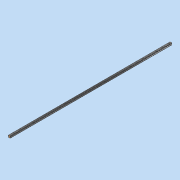
# Autodesk Inventor part: HGR20 THANH TRUOT
Saved by Autodesk Inventor 2021 (Build 250183000, 183)
## iProperties
Created: 2021-09-26
Part Number: HGR20 THANH TRUOT
Material: Generic
Document SubType Name: Modeling
Designer: 41601100
Density: 1 g/cm^3
Appearance: Default
Author: 41601100
Autodesk Inventor part; units mm, degrees
ref_plane "YZ Plane" through (0, 0, 0) normal (1, 0, 0) x (0, 1, 0)
ref_plane "XZ Plane" through (0, 0, 0) normal (0, 1, 0) x (-1, 0, 0)
ref_plane "XY Plane" through (0, 0, 0) normal (0, 0, 1) x (1, 0, 0)
sketch "Sketch1" plane through (0, 0, 0) normal (0, 0, 1) x (1, 0, 0)
  arc A0 (-9.7071, -9.6314) -> (-10, -10.3385) centre (-9, -10.3385) ccw
  line L0 (-10, -10.3385) -> (-10, -13)
  line L1 (-10, -13) -> (-9, -14)
  line L2 (-9, -14) -> (9, -14)
  line L3 (9, -14) -> (10, -13)
  line L4 (10, -13) -> (10, -10.3385)
  arc A1 (10, -10.3385) -> (9.7071, -9.6314) centre (9, -10.3385) ccw
  line L5 (9.7071, -9.6314) -> (6.8929, -6.8172)
  arc A2 (6.6, -6.1101) -> (6.8929, -6.8172) centre (7.6, -6.1101) ccw
  line L6 (6.6, -6.1101) -> (6.6, -4.5499)
  arc A3 (6.8929, -3.8428) -> (6.6, -4.5499) centre (7.6, -4.5499) ccw
  line L7 (6.8929, -3.8428) -> (7.6302, -3.1056)
  arc A4 (7.6302, -3.1056) -> (7.8468, -2.7675) centre (7.3529, -2.6895) ccw
  arc A5 (9.4318, -1.1825) -> (7.8468, -2.7675) centre (9.8106, -3.1463) ccw
  arc A6 (9.4318, -1.1825) -> (9.6906, -1.0451) centre (9.3371, -0.6915) ccw
  line L8 (9.6906, -1.0451) -> (9.8536, -0.8822)
  arc A7 (9.8536, -0.8822) -> (10, -0.5286) centre (9.5, -0.5286) ccw
  line L9 (10, -0.5286) -> (10, 0.5286)
  arc A8 (10, 0.5286) -> (9.8536, 0.8822) centre (9.5, 0.5286) ccw
  line L10 (9.8536, 0.8822) -> (9.6906, 1.0451)
  arc A9 (9.6906, 1.0451) -> (9.4224, 1.1941) centre (9.3254, 0.7036) ccw
  arc A10 (7.8482, 2.768) -> (9.4224, 1.1941) centre (9.8101, 3.1561) ccw
  arc A11 (7.8482, 2.768) -> (7.6325, 3.1032) centre (7.3547, 2.6875) ccw
  line L11 (7.6325, 3.1032) -> (7.2357, 3.5)
  line L12 (7.2357, 3.5) -> (-7.2357, 3.5)
  line L13 (-7.2357, 3.5) -> (-7.6325, 3.1032)
  arc A12 (-7.6325, 3.1032) -> (-7.8482, 2.768) centre (-7.3547, 2.6875) ccw
  arc A13 (-9.4224, 1.1941) -> (-7.8482, 2.768) centre (-9.8101, 3.1561) ccw
  arc A14 (-9.4224, 1.1941) -> (-9.6906, 1.0451) centre (-9.3254, 0.7036) ccw
  line L14 (-9.6906, 1.0451) -> (-9.8536, 0.8822)
  arc A15 (-9.8536, 0.8822) -> (-10, 0.5286) centre (-9.5, 0.5286) ccw
  line L15 (-10, 0.5286) -> (-10, -0.5286)
  arc A16 (-10, -0.5286) -> (-9.8536, -0.8822) centre (-9.5, -0.5286) ccw
  line L16 (-9.8536, -0.8822) -> (-9.6906, -1.0451)
  arc A17 (-9.6906, -1.0451) -> (-9.4318, -1.1825) centre (-9.3371, -0.6915) ccw
  arc A18 (-7.8468, -2.7675) -> (-9.4318, -1.1825) centre (-9.8106, -3.1463) ccw
  arc A19 (-7.8468, -2.7675) -> (-7.6302, -3.1056) centre (-7.3529, -2.6895) ccw
  line L17 (-7.6302, -3.1056) -> (-6.8929, -3.8428)
  arc A20 (-6.6, -4.5499) -> (-6.8929, -3.8428) centre (-7.6, -4.5499) ccw
  line L18 (-6.6, -4.5499) -> (-6.6, -6.1101)
  arc A21 (-6.8929, -6.8172) -> (-6.6, -6.1101) centre (-7.6, -6.1101) ccw
  line L19 (-6.8929, -6.8172) -> (-9.7071, -9.6314)
  point P0 (0, 0)
  point P1 (0, 0)
  constraints: 44 point on circle, 40 end point, 22 centre point
extrude "Extrusion1" add sketch "Sketch1" along normal blind 1500
sketch "Sketch2" plane through (-7.2357, 3.5, 1500) normal (0, 1, 0) x (1, 0, 0)
  line L0 (14.4714, 1500) -> (0, 1500) projected
  line L1 (0, 1500) -> (0, 0) projected
  line L2 (14.4714, 0) -> (0, 0) projected
  line L3 (14.4714, 1500) -> (14.4714, 0) projected
  circle A0 centre (7.2357, 1480) radius 4.75
  circle A1 centre (7.2357, 1480) radius 3
  circle A2 centre (7.2357, 1420) radius 4.75
  circle A3 centre (7.2357, 1420) radius 3
  circle A4 centre (7.2357, 1360) radius 4.75
  circle A5 centre (7.2357, 1360) radius 3
  circle A6 centre (7.2357, 1300) radius 4.75
  circle A7 centre (7.2357, 1300) radius 3
  circle A8 centre (7.2357, 1240) radius 4.75
  circle A9 centre (7.2357, 1240) radius 3
  circle A10 centre (7.2357, 1180) radius 4.75
  circle A11 centre (7.2357, 1180) radius 3
  circle A12 centre (7.2357, 1120) radius 4.75
  circle A13 centre (7.2357, 1120) radius 3
  circle A14 centre (7.2357, 1060) radius 4.75
  circle A15 centre (7.2357, 1060) radius 3
  circle A16 centre (7.2357, 1000) radius 4.75
  circle A17 centre (7.2357, 1000) radius 3
  circle A18 centre (7.2357, 940) radius 4.75
  circle A19 centre (7.2357, 940) radius 3
  circle A20 centre (7.2357, 880) radius 4.75
  circle A21 centre (7.2357, 880) radius 3
  circle A22 centre (7.2357, 820) radius 4.75
  circle A23 centre (7.2357, 820) radius 3
  circle A24 centre (7.2357, 760) radius 4.75
  circle A25 centre (7.2357, 760) radius 3
  circle A26 centre (7.2357, 700) radius 4.75
  circle A27 centre (7.2357, 700) radius 3
  circle A28 centre (7.2357, 640) radius 4.75
  circle A29 centre (7.2357, 640) radius 3
  circle A30 centre (7.2357, 580) radius 4.75
  circle A31 centre (7.2357, 580) radius 3
  circle A32 centre (7.2357, 520) radius 4.75
  circle A33 centre (7.2357, 520) radius 3
  circle A34 centre (7.2357, 460) radius 4.75
  circle A35 centre (7.2357, 460) radius 3
  circle A36 centre (7.2357, 400) radius 4.75
  circle A37 centre (7.2357, 400) radius 3
  circle A38 centre (7.2357, 340) radius 4.75
  circle A39 centre (7.2357, 340) radius 3
  circle A40 centre (7.2357, 280) radius 4.75
  circle A41 centre (7.2357, 280) radius 3
  circle A42 centre (7.2357, 220) radius 4.75
  circle A43 centre (7.2357, 220) radius 3
  circle A44 centre (7.2357, 160) radius 4.75
  circle A45 centre (7.2357, 160) radius 3
  circle A46 centre (7.2357, 100) radius 4.75
  circle A47 centre (7.2357, 100) radius 3
  circle A48 centre (7.2357, 40) radius 4.75
  circle A49 centre (7.2357, 40) radius 3
  point P0 (7.2357, 1500)
  dimension "d3" = 9.5
  dimension "d4" = 6
  dimension "d6" = 9.5
  dimension "d7" = 6
  dimension "d9" = 9.5
  dimension "d10" = 6
  dimension "d12" = 9.5
  dimension "d13" = 6
  dimension "d15" = 9.5
  dimension "d16" = 6
  dimension "d18" = 9.5
  dimension "d19" = 6
  dimension "d21" = 9.5
  dimension "d22" = 6
  dimension "d24" = 9.5
  dimension "d25" = 6
  dimension "d27" = 9.5
  dimension "d28" = 6
  dimension "d30" = 9.5
  dimension "d31" = 6
  dimension "d33" = 9.5
  dimension "d34" = 6
  dimension "d36" = 9.5
  dimension "d37" = 6
  dimension "d39" = 9.5
  dimension "d40" = 6
  dimension "d42" = 9.5
  dimension "d43" = 6
  dimension "d45" = 9.5
  dimension "d46" = 6
  dimension "d48" = 9.5
  dimension "d49" = 6
  dimension "d51" = 9.5
  dimension "d52" = 6
  dimension "d54" = 9.5
  dimension "d55" = 6
  dimension "d57" = 9.5
  dimension "d58" = 6
  dimension "d60" = 9.5
  dimension "d61" = 6
  dimension "d63" = 9.5
  dimension "d64" = 6
  dimension "d66" = 9.5
  dimension "d67" = 6
  dimension "d69" = 9.5
  dimension "d70" = 6
  dimension "d72" = 9.5
  dimension "d73" = 6
  dimension "d75" = 9.5
  dimension "d76" = 6
  constraints: 50 centre point, 25 coincident
  measures "d3" diameter of A0
  measures "d4" diameter of A1
  measures "d6" diameter of A2
  measures "d7" diameter of A3
  measures "d9" diameter of A4
  measures "d10" diameter of A5
  measures "d12" diameter of A6
  measures "d13" diameter of A7
  measures "d15" diameter of A8
  measures "d16" diameter of A9
  measures "d18" diameter of A10
  measures "d19" diameter of A11
  measures "d21" diameter of A12
  measures "d22" diameter of A13
  measures "d24" diameter of A14
  measures "d25" diameter of A15
  measures "d27" diameter of A16
  measures "d28" diameter of A17
  measures "d30" diameter of A18
  measures "d31" diameter of A19
  measures "d33" diameter of A20
  measures "d34" diameter of A21
  measures "d36" diameter of A22
  measures "d37" diameter of A23
  measures "d39" diameter of A24
  measures "d40" diameter of A25
  measures "d42" diameter of A26
  measures "d43" diameter of A27
  measures "d45" diameter of A28
  measures "d46" diameter of A29
  measures "d48" diameter of A30
  measures "d49" diameter of A31
  measures "d51" diameter of A32
  measures "d52" diameter of A33
  measures "d54" diameter of A34
  measures "d55" diameter of A35
  measures "d57" diameter of A36
  measures "d58" diameter of A37
  measures "d60" diameter of A38
  measures "d61" diameter of A39
  measures "d63" diameter of A40
  measures "d64" diameter of A41
  measures "d66" diameter of A42
  measures "d67" diameter of A43
  measures "d69" diameter of A44
  measures "d70" diameter of A45
  measures "d72" diameter of A46
  measures "d73" diameter of A47
  measures "d75" diameter of A48
  measures "d76" diameter of A49
extrude "Extrusion2" cut sketch "Sketch2" against normal blind 30 contours A1 | A3 | A5 | A7 | A9 | A11 | A13 | A15 | A17 | A19 | A21 | A23 | A25 | A27 | A29 | A31 | A35 | A37 | A39 | A41 | A43 | A45 | A47 | A49
extrude "Extrusion3" cut sketch "Sketch2" against normal blind 8.4 contours A0 | A2 | A4 | A6 | A8 | A10 | A11 | A12 | A14 | A16 | A18 | A20 | A24 | A26 | A28 | A30 | A32 | A34 | A36 | A38 | A40 | A42 | A44 | A46 | A48
sketch "Sketch3" plane through (0, 0, 1500) normal (0, 0, 1) x (1, 0, 0)
  line L0 (9.6906, -1.0451) -> (9.8536, -0.8822) projected
  arc A0 (9.8536, -0.8822) -> (10, -0.5286) centre (9.5, -0.5286) ccw projected
  line L1 (10, -0.5286) -> (10, 0.5286) projected
  arc A1 (10, 0.5286) -> (9.8536, 0.8822) centre (9.5, 0.5286) ccw projected
  line L2 (9.8536, 0.8822) -> (9.6906, 1.0451) projected
  arc A2 (9.6906, 1.0451) -> (9.4224, 1.1941) centre (9.3254, 0.7036) ccw projected
  arc A3 (7.8482, 2.768) -> (9.4224, 1.1941) centre (9.8101, 3.1561) ccw projected
  arc A4 (7.8482, 2.768) -> (7.6325, 3.1032) centre (7.3547, 2.6875) ccw projected
  line L3 (7.6325, 3.1032) -> (7.2357, 3.5) projected
  line L4 (7.2357, 3.5) -> (-7.2357, 3.5) projected
  line L5 (-7.2357, 3.5) -> (-7.6325, 3.1032) projected
  arc A5 (-7.6325, 3.1032) -> (-7.8482, 2.768) centre (-7.3547, 2.6875) ccw projected
  arc A6 (-9.4224, 1.1941) -> (-7.8482, 2.768) centre (-9.8101, 3.1561) ccw projected
  arc A7 (-9.4224, 1.1941) -> (-9.6906, 1.0451) centre (-9.3254, 0.7036) ccw projected
  line L6 (-9.6906, 1.0451) -> (-9.8536, 0.8822) projected
  arc A8 (-9.8536, 0.8822) -> (-10, 0.5286) centre (-9.5, 0.5286) ccw projected
  line L7 (-10, 0.5286) -> (-10, -0.5286) projected
  arc A9 (-10, -0.5286) -> (-9.8536, -0.8822) centre (-9.5, -0.5286) ccw projected
  line L8 (-9.8536, -0.8822) -> (-9.6906, -1.0451) projected
  arc A10 (-9.6906, -1.0451) -> (-9.4318, -1.1825) centre (-9.3371, -0.6915) ccw projected
  arc A11 (-7.8468, -2.7675) -> (-9.4318, -1.1825) centre (-9.8106, -3.1463) ccw projected
  arc A12 (-7.8468, -2.7675) -> (-7.6302, -3.1056) centre (-7.3529, -2.6895) ccw projected
  line L9 (-7.6302, -3.1056) -> (-6.8929, -3.8428) projected
  arc A13 (-6.6, -4.5499) -> (-6.8929, -3.8428) centre (-7.6, -4.5499) ccw projected
  line L10 (-6.6, -4.5499) -> (-6.6, -6.1101) projected
  arc A14 (-6.8929, -6.8172) -> (-6.6, -6.1101) centre (-7.6, -6.1101) ccw projected
  line L11 (-6.8929, -6.8172) -> (-9.7071, -9.6314) projected
  arc A15 (-9.7071, -9.6314) -> (-10, -10.3385) centre (-9, -10.3385) ccw projected
  line L12 (-10, -10.3385) -> (-10, -13) projected
  line L13 (-10, -13) -> (-9, -14) projected
  line L14 (-9, -14) -> (9, -14) projected
  line L15 (9, -14) -> (10, -13) projected
  line L16 (10, -13) -> (10, -10.3385) projected
  arc A16 (10, -10.3385) -> (9.7071, -9.6314) centre (9, -10.3385) ccw projected
  line L17 (9.7071, -9.6314) -> (6.8929, -6.8172) projected
  arc A17 (6.6, -6.1101) -> (6.8929, -6.8172) centre (7.6, -6.1101) ccw projected
  line L18 (6.6, -6.1101) -> (6.6, -4.5499) projected
  arc A18 (6.8929, -3.8428) -> (6.6, -4.5499) centre (7.6, -4.5499) ccw projected
  line L19 (6.8929, -3.8428) -> (7.6302, -3.1056) projected
  arc A19 (7.6302, -3.1056) -> (7.8468, -2.7675) centre (7.3529, -2.6895) ccw projected
  arc A20 (9.4318, -1.1825) -> (7.8468, -2.7675) centre (9.8106, -3.1463) ccw projected
  arc A21 (9.4318, -1.1825) -> (9.6906, -1.0451) centre (9.3371, -0.6915) ccw projected
  line L20 (-4.75, 3.5) -> (4.75, 3.5) projected
  line L21 (0, 3.5) -> (0, -14)
  point P0 (0, 0)
  constraints: 2 end point, 2 midpoint
sketch "Sketch4" plane through (0, 0, 0) normal (0, 0, -1) x (-1, 0, 0)
  line L0 (-9.6906, -1.0451) -> (-9.8536, -0.8822) projected
  arc A0 (-9.6906, -1.0451) -> (-9.4318, -1.1825) centre (-9.3371, -0.6915) ccw projected
  arc A1 (-7.8468, -2.7675) -> (-9.4318, -1.1825) centre (-9.8106, -3.1463) ccw projected
  arc A2 (-7.8468, -2.7675) -> (-7.6302, -3.1056) centre (-7.3529, -2.6895) ccw projected
  line L1 (-6.8929, -3.8428) -> (-7.6302, -3.1056) projected
  arc A3 (-6.6, -4.5499) -> (-6.8929, -3.8428) centre (-7.6, -4.5499) ccw projected
  line L2 (-6.6, -6.1101) -> (-6.6, -4.5499) projected
  arc A4 (-6.8929, -6.8172) -> (-6.6, -6.1101) centre (-7.6, -6.1101) ccw projected
  line L3 (-9.7071, -9.6314) -> (-6.8929, -6.8172) projected
  arc A5 (-9.7071, -9.6314) -> (-10, -10.3385) centre (-9, -10.3385) ccw projected
  line L4 (-10, -13) -> (-10, -10.3385) projected
  line L5 (-9, -14) -> (-10, -13) projected
  line L6 (9, -14) -> (-9, -14) projected
  line L7 (10, -13) -> (9, -14) projected
  line L8 (10, -10.3385) -> (10, -13) projected
  arc A6 (10, -10.3385) -> (9.7071, -9.6314) centre (9, -10.3385) ccw projected
  line L9 (6.8929, -6.8172) -> (9.7071, -9.6314) projected
  arc A7 (6.6, -6.1101) -> (6.8929, -6.8172) centre (7.6, -6.1101) ccw projected
  line L10 (6.6, -4.5499) -> (6.6, -6.1101) projected
  arc A8 (6.8929, -3.8428) -> (6.6, -4.5499) centre (7.6, -4.5499) ccw projected
  line L11 (7.6302, -3.1056) -> (6.8929, -3.8428) projected
  arc A9 (7.6302, -3.1056) -> (7.8468, -2.7675) centre (7.3529, -2.6895) ccw projected
  arc A10 (9.4318, -1.1825) -> (7.8468, -2.7675) centre (9.8106, -3.1463) ccw projected
  arc A11 (9.4318, -1.1825) -> (9.6906, -1.0451) centre (9.3371, -0.6915) ccw projected
  line L12 (9.8536, -0.8822) -> (9.6906, -1.0451) projected
  arc A12 (9.8536, -0.8822) -> (10, -0.5286) centre (9.5, -0.5286) ccw projected
  line L13 (10, 0.5286) -> (10, -0.5286) projected
  arc A13 (10, 0.5286) -> (9.8536, 0.8822) centre (9.5, 0.5286) ccw projected
  line L14 (9.6906, 1.0451) -> (9.8536, 0.8822) projected
  arc A14 (9.6906, 1.0451) -> (9.4224, 1.1941) centre (9.3254, 0.7036) ccw projected
  arc A15 (7.8482, 2.768) -> (9.4224, 1.1941) centre (9.8101, 3.1561) ccw projected
  arc A16 (7.8482, 2.768) -> (7.6325, 3.1032) centre (7.3547, 2.6875) ccw projected
  line L15 (7.2357, 3.5) -> (7.6325, 3.1032) projected
  line L16 (-7.2357, 3.5) -> (7.2357, 3.5) projected
  line L17 (-7.6325, 3.1032) -> (-7.2357, 3.5) projected
  arc A17 (-7.6325, 3.1032) -> (-7.8482, 2.768) centre (-7.3547, 2.6875) ccw projected
  arc A18 (-9.4224, 1.1941) -> (-7.8482, 2.768) centre (-9.8101, 3.1561) ccw projected
  arc A19 (-9.4224, 1.1941) -> (-9.6906, 1.0451) centre (-9.3254, 0.7036) ccw projected
  line L18 (-9.8536, 0.8822) -> (-9.6906, 1.0451) projected
  arc A20 (-9.8536, 0.8822) -> (-10, 0.5286) centre (-9.5, 0.5286) ccw projected
  line L19 (-10, -0.5286) -> (-10, 0.5286) projected
  arc A21 (-10, -0.5286) -> (-9.8536, -0.8822) centre (-9.5, -0.5286) ccw projected
  line L20 (0, 3.5) -> (0, -14)
  point P0 (0, 0)
  constraints: 2 end point, 2 midpoint
body "Solid1"
